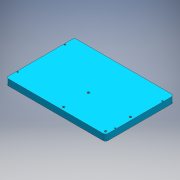
# Autodesk Inventor part: sampleHolderBase
Saved by Autodesk Inventor 2016 (Build 200138000, 138)
## iProperties
Created: 2016-03-01
Part Number: sampleHolderBase
Material: Generic
Document SubType Name: Modeling
Designer: sims01
Density: 1 g/cm^3
Appearance: Default
Author: sims01
Autodesk Inventor part; units mm, degrees
ref_plane "YZ Plane" through (0, 0, 0) normal (1, 0, 0) x (0, 1, 0)
ref_plane "XZ Plane" through (0, 0, 0) normal (0, 1, 0) x (-1, 0, 0)
ref_plane "XY Plane" through (0, 0, 0) normal (0, 0, 1) x (1, 0, 0)
sketch "Sketch1" plane through (0, 0, 0) normal (0, 0, 1) x (1, 0, 0)
  line L0 (-76, 55) -> (76, 55)
  line L1 (80, 51) -> (80, -51)
  line L2 (76, -55) -> (-76, -55)
  line L3 (-80, -51) -> (-80, 51)
  arc A0 (-76, 55) -> (-80, 51) centre (-76, 51) ccw
  arc A1 (-80, -51) -> (-76, -55) centre (-76, -51) ccw
  arc A2 (76, -55) -> (80, -51) centre (76, -51) ccw
  arc A3 (80, 51) -> (76, 55) centre (76, 51) ccw
  point P0 (0, 0)
  point P1 (-80, 55)
  point P2 (80, -55)
  point P3 (80, 55)
  dimension "d0" = 160
  dimension "d1" = 80
  dimension "d2" = 110
  dimension "d3" = 55
  dimension "d4" = 4
  constraints: 8 end point, 8 point on circle, 8 tangent, 6 point on line, 4 centre point, 3 equal radius, 2 parallel, 1 horizontal, 1 perpendicular
  measures "d0" distance of point (-80, 55) point (80, 55)
  measures "d1" distance from line of point (0, 0) L1
  measures "d2" distance of point (80, 55) point (80, -55)
  measures "d3" distance from line of point (0, 0) L0
  measures "d4" radius of A0
extrude "baseExtrusion" add sketch "Sketch1" along normal blind 10
sketch "Sketch2" plane through (0, 0, 10) normal (0, 0, 1) x (1, 0, 0)
  line L0 (-76, -55) -> (76, -55) projected
  point P0 (0, 0)
  point P1 (-78.3, 38)
  point P2 (78.3, 38)
  point P3 (-78.3, -38)
  point P4 (78.3, -38)
  dimension "d7" = 156.6
  dimension "d8" = 78.3
  dimension "d9" = 76
  dimension "d18" = 38
  constraints: 2 horizontal alignment, 2 vertical alignment
  measures "d7" distance of point (-78.3, 38) point (78.3, 38)
  measures "d8" horizontal distance of point (0, 0) point (78.3, 38)
  measures "d9" distance of point (-78.3, -38) point (-78.3, 38)
  measures "d18" vertical distance of point (0, 0) point (-78.3, 38)
hole "baseXYStageMountingHoles" at (-78.3, 38, 10) at (78.3, 38, 10) at (-78.3, -38, 10) at (78.3, -38, 10) direction (0, 0, -1) diameter 2.013 end through all thread size "M2.5x0.45" class "6H" standard "ISO Metric profile"
sketch "Sketch4" plane through (0, 0, 10) normal (0, 0, 1) x (1, 0, 0)
  line L0 (-76, -55) -> (76, -55) projected
  line L1 (80, -51) -> (80, 51) projected
  point P0 (0, 0)
  point P1 (75, -50)
  point P2 (75, -10)
  point P3 (7.5, -50)
  point P4 (7.5, -10)
  dimension "d30" = 40
  dimension "d31" = 67.5
  dimension "d32" = 5
  dimension "d33" = 5
  constraints: 2 horizontal alignment, 2 vertical alignment
  measures "d30" distance of point (75, -50) point (75, -10)
  measures "d31" distance of point (75, -10) point (7.5, -10)
  measures "d32" distance from line of L0 point (7.5, -50)
  measures "d33" distance from line of L1 point (75, -50)
hole "Hole3" at (75, -50, 10) at (75, -10, 10) at (7.5, -50, 10) at (7.5, -10, 10) direction (0, 0, -1) diameter 3.242 depth 11.8 tip angle 118 thread size "M4x0.7" class "6H" standard "ISO Metric profile"
equation "\"d0\" = sampleHolderBaseX"
equation "\"d1\" = 0.5 * d0"
equation "\"d2\" = sampleHolderBaseY"
equation "\"d3\" = 0.5 * d2"
equation "\"d4\" = sampleHolderFilletRadius"
equation "\"d5\" = sampleHolderBaseZ"
equation "\"d7\" = sampleHolderM25MountingX"
equation "\"d8\" = 0.5 * d7"
equation "\"d9\" = sampleHolderM25MountingY"
equation "\"d18\" = 0.5 * d9"
equation "\"sampleHolderBaseX\" = 160"
equation "\"sampleHolderBaseY\" = 110"
equation "\"sampleHolderBaseZ\" = 10"
equation "\"sampleHolderM25MountingY\" = 76"
equation "\"sampleHolderM25MountingX\" = 156.6"
equation "\"sampleHolderFilletRadius\" = 4"
equation "\"specificSampleHolderBaseTroughDepth\" = 5"
equation "\"specificSampleHolderMountXseparation_1\" = 155"
equation "\"specificSampleHolderMountYseparation_1\" = 25"
equation "\"specificSampleHolderBaseX_excess\" = 15.5"
equation "\"specificSampleHolderMountLHSseparation\" = 41"
equation "\"specificSampleHolderBaseTroughDiameter\" = 5"
equation "\"specificSampleHolderBaseX\" = 135"
equation "\"sampleHolderEnclosureStiltY\" = 41"
equation "\"specificSampleHolderBaseStiltHeight\" = 4"
equation "\"sampleHolderEnclosureExcessX\" = 15"
equation "\"sampleHolderEnclosureExcessY\" = 15"
equation "\"sampleHolderEnclosureStiltX\" = 136"
equation "\"sampleHolderEnclosureStiltDiameter\" = 3"
equation "\"sampleHolderEnclosureWallThickness_x\" = 5"
equation "\"sampleHolderEnclosureWallThickness_y2\" = 5"
equation "\"glassWindowApertureExcess\" = 5"
equation "\"glassWindowApertureHeightAboveBase\" = 5"
equation "\"glassWindowDistanceFromOuterWall\" = 1"
equation "\"glassWindowActX\" = 122.5"
equation "\"glassWindowActY\" = 32.5"
equation "\"glassWindowThickness\" = 2"
equation "\"sampleHolderLidExcessX\" = 15"
equation "\"sampleHolderLidThickness\" = 5"
equation "\"objectiveMaxDiam\" = 39"
equation "\"sampleHolderLidObjectiveExcess\" = 2"
equation "\"FilipeSampleBaseSecondExtrusionHeight\" = 5"
equation "\"FilipeSampleAngle\" = 10deg"
equation "\"specificSampleHolderBaseZ_2\" = 5"
body "Solid1"
